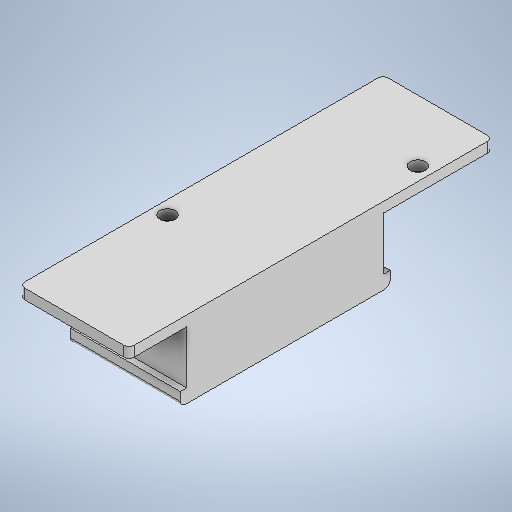
# Autodesk Inventor part: Platte 12V modul
Saved by Autodesk Inventor 2025.2 (Build 292293000, 293)
## iProperties
Created: 2025-03-23
Part Number: Platte 12V modul
Material: Generisch
Document SubType Name: Modeling
Designer: Quatana
Density: 1 g/cm^3
Appearance: Vorgabe
Author: Quatana
## iProperties of the stored document Relais_Platte_3D-Druck.ipt
Created: 2025-03-23
Part Number: Relais_Platte_3D-Druck
Material: Generisch
Document SubType Name: Modeling
Designer: Quatana
Density: 1 g/cm^3
Appearance: Vorgabe
Author: Quatana
Autodesk Inventor part; units mm, degrees
ref_plane "YZ Plane" through (0, 0, 0) normal (1, 0, 0) x (0, 1, 0)
ref_plane "XZ Plane" through (0, 0, 0) normal (0, 1, 0) x (-1, 0, 0)
ref_plane "XY Plane" through (0, 0, 0) normal (0, 0, 1) x (1, 0, 0)
sketch "Skizze1" plane through (0, 0, 0) normal (0, 0, 1) x (1, 0, 0)
  line L0 (-10.7, -35.5) -> (10.7, -35.5)
  line L1 (10.7, -35.5) -> (10.7, 35.5)
  line L2 (10.7, 35.5) -> (-10.7, 35.5)
  line L3 (-10.7, 35.5) -> (-10.7, -35.5)
  line L4 (-10.7, -35.5) -> (10.7, 35.5) construction
  line L5 (10.7, -35.5) -> (-10.7, 35.5) construction
  point P0 (0, 0)
  dimension "d0" = 21.4
  dimension "d1" = 71
  constraints: 12 end point, 2 midpoint, 2 parallel, 1 horizontal, 1 perpendicular
  measures "d0" distance of L2.end L1.end
  measures "d1" distance of L1.end L0.end
extrude "Extrusion1" add sketch "Skizze1" along normal blind 2
sketch "Skizze2" plane through (0, 0, 2) normal (0, 0, 1) x (1, 0, 0)
  line L0 (10.7, 35.5) -> (-10.7, 35.5) projected
  line L1 (0, 35.5) -> (0, 32.4568) construction
  line L2 (-3.3034, 0) -> (2.2681, 0) construction
  line L3 (-10.7, 35.5) -> (-10.7, -35.5) construction
  circle A0 centre (8.08, 23.5) radius 1.5
  circle A1 centre (-8.08, -9.2) radius 1.5
  line L4 (9.58, 23.5) -> (10.7, 23.5)
  line L5 (10.7, -35.5) -> (10.7, 35.5) projected
  line L6 (-9.58, -9.2) -> (-10.7, -9.2)
  point P0 (0, 0)
  point P1 (10.14, 23.5)
  point P2 (-10.14, -9.2)
  dimension "d18" = 3
  dimension "d19" = 3
  dimension "d21" = 1.12
  dimension "d22" = 1.12
  dimension "d23" = 32.7
  dimension "d24" = 12
  constraints: 8 end point, 4 horizontal alignment, 3 horizontal, 3 midpoint, 2 point on line, 1 vertical, 4 other
  measures "d21" distance of L4.start L4.end
  measures "d22" distance of L6.start L6.end
  measures "d23" vertical distance of point (8.08, 23.5) point (-8.08, -9.2)
  measures "d24" distance from line of L0 point (8.08, 23.5)
extrude "Extrusion2" cut sketch "Skizze2" against normal blind 4
sketch "Skizze3" plane through (0, 0, 0) normal (0, 0, -1) x (-1, 0, 0)
  line L0 (10.7, 35.5) -> (10.7, -35.5) projected
  line L1 (-10.7, -25.5) -> (10.7, -25.5)
  line L2 (10.7, -25.5) -> (10.7, 15.5)
  line L3 (10.7, 15.5) -> (-10.7, 15.5)
  line L4 (-10.7, 15.5) -> (-10.7, -25.5)
  line L5 (-10.7, -25.5) -> (10.7, 15.5) construction
  line L6 (10.7, -25.5) -> (-10.7, 15.5) construction
  line L7 (10.7, -35.5) -> (-10.7, -35.5) projected
  line L8 (-10.7, -35.5) -> (-10.7, 35.5) projected
  point P0 (0, -5)
  point P1 (10.7, -25.5)
  dimension "d9" = 41
  dimension "d17" = 10
  constraints: 12 end point, 2 midpoint, 2 parallel, 1 horizontal, 1 perpendicular, 1 point on line, 1 vertical alignment
  measures "d9" distance between parallel lines of L1 L3
  measures "d17" distance between parallel lines of L7 L1
extrude "Extrusion3" add sketch "Skizze3" along normal blind 13 contours L0 L1 L4 L3
sketch "Skizze4" plane through (-10.7, -35.5, 2) normal (-1, 0, 0) x (0, 0, 1)
  line L0 (-2, 10) -> (-15, 10) projected
  line L1 (-12.32, 10) -> (-2, 10)
  line L2 (-2, 10) -> (-2, 11.25)
  line L3 (-2, 11.25) -> (-12.32, 11.25)
  line L4 (-12.32, 11.25) -> (-12.32, 10)
  line L5 (-15, 10) -> (-15, 51) projected
  line L6 (-4.404, 30.5) -> (2.981, 30.5) construction
  line L7 (-2, 51) -> (-15, 51)
  line L8 (-2, 51) -> (-2, 49.75)
  line L9 (-2, 49.75) -> (-12.32, 49.75)
  line L10 (-12.32, 49.75) -> (-12.32, 51)
  line L11 (-2, 10) -> (-12.32, 10)
  point P0 (-2, 35.5)
  point P1 (-12.32, 10.625)
  dimension "d12" = 2.68
  dimension "d13" = 1.25
  constraints: 20 end point, 5 symmetric about line, 3 point on line, 2 horizontal, 2 parallel, 1 collinear, 1 midpoint, 1 perpendicular
  measures "d12" distance from line of L5 point (-12.32, 10.625)
  measures "d13" distance between parallel lines of L3 L0
extrude "Extrusion4" cut sketch "Skizze4" against normal through all
fillet "Rundung1" radius 1 6 edges at (-10.7, -35.5, 1) (10.7, -35.5, 1) (10.7, 35.5, 1) (-10.7, 35.5, 1) (0, 15.5, -13) (0, -25.5, -13)
sketch "Skizze5" plane through (-10.7, -24.25, -10.32) normal (-1, 0, 0) x (0, 0, 1)
  line L0 (12.32, 16.55) -> (12.32, 13.55) projected
  line L1 (10.32, 13.55) -> (10.32, 16.55) projected
  line L2 (10.32, 13.55) -> (10.32, 16.55) projected
  line L3 (12.32, 16.55) -> (12.32, 13.55) projected
  circle A0 centre (8.82, 15.05) radius 1.5
  point P0 (10.32, 24.25)
  point P1 (10.32, 15.05)
  dimension "d25" = 3
  constraints: 1 horizontal alignment, 1 midpoint, 2 other
loft "Erhebung2" cut profiles "Skizze5" section 2 edges at (-9.58, -9.2, 0)
